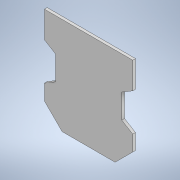
# Autodesk Inventor part: BaseCarro
Saved by Autodesk Inventor 2021 (Build 250183000, 183)
## iProperties
Created: 2021-02-05
Part Number: BaseCarro
Material: Genérico
Document SubType Name: Modeling
Designer: jaime
Density: 1 g/cm^3
Appearance: Valor por defecto
Author: jaime
Autodesk Inventor part; units mm, degrees
ref_plane "YZ Plane" through (0, 0, 0) normal (1, 0, 0) x (0, 1, 0)
ref_plane "XZ Plane" through (0, 0, 0) normal (0, 1, 0) x (-1, 0, 0)
ref_plane "XY Plane" through (0, 0, 0) normal (0, 0, 1) x (1, 0, 0)
sketch "Boceto1" plane through (0, 0, 0) normal (0, 0, 1) x (1, 0, 0)
  line L0 (0, 0) -> (-200, 0)
  line L1 (-200, 0) -> (-200, -120)
  line L2 (-200, -120) -> (-150, -150)
  line L3 (-150, -150) -> (-150, -260)
  line L4 (-150, -260) -> (-200, -290)
  line L5 (-200, -290) -> (-200, -360)
  line L6 (-200, -360) -> (-120, -440)
  line L7 (-120, -440) -> (0, -440)
  line L8 (0, -440) -> (0, 0) construction
  line L9 (0, 0) -> (200, 0)
  line L10 (200, 0) -> (200, -120)
  line L11 (200, -120) -> (150, -150)
  line L12 (150, -150) -> (150, -260)
  line L13 (150, -260) -> (200, -290)
  line L14 (200, -290) -> (200, -360)
  line L15 (200, -360) -> (120, -440)
  line L16 (120, -440) -> (0, -440)
  dimension "d0" = 120
  dimension "d1" = 70
  dimension "d2" = 110
  dimension "d3" = 200
  dimension "d8" = 120
  dimension "d9" = 80
  dimension "d13" = 150
  dimension "d17" = 80
  dimension "d18" = 30
  dimension "d19" = 30
  constraints: 34 end point, 7 symmetric about line, 2 horizontal, 2 perpendicular, 1 parallel, 1 vertical
  measures "d0" distance of L0.end L1.end
  measures "d1" distance of L4.end L5.end
  measures "d2" distance of L2.end L3.end
  measures "d3" distance of L0.start L0.end
  measures "d8" distance of L6.end L7.end
  measures "d9" horizontal distance of L5.end L6.end
  measures "d13" distance between parallel lines of L3 L8
  measures "d17" horizontal distance of L5.end L6.end
  measures "d18" vertical distance of L3.end L4.end
  measures "d19" vertical distance of L1.end L2.end
extrude "Extrusión1" add sketch "Boceto1" along normal mid plane 12.55
